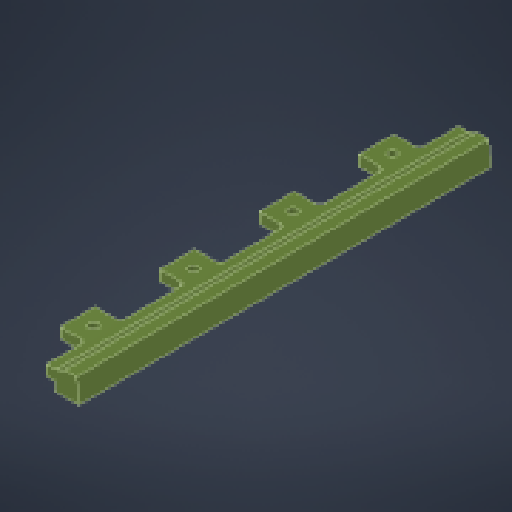
# Autodesk Inventor part: plaski_plog
Saved by Autodesk Inventor 2023 (Build 270158000, 158)
## iProperties
Created: 2024-06-19
Part Number: plaski_plog
Material: PC/ABS Plastic
Document SubType Name: Modeling
Designer: szymo
Density: 1.1 g/cm^3
Appearance: Dark Olive
Mass: 23.2841 g
Surface Area: 101.304 cm^2
Volume: 21.1673 cm^3
Author: szymo
Autodesk Inventor part; units mm, degrees
ref_plane "YZ Plane" through (0, 0, 0) normal (1, 0, 0) x (0, 1, 0)
ref_plane "XZ Plane" through (0, 0, 0) normal (0, 1, 0) x (-1, 0, 0)
sketch "Sketch1" plane through (0, 0, 0) normal (0, 0, 1) x (1, 0, 0)
  line L0 (-60.5213, -2.6863) -> (-60.5213, -7.1863) projected
  line L1 (-69.5213, -2.6863) -> (-60.5213, -2.6863) projected
  line L2 (-69.5213, -7.1863) -> (-69.5213, -2.6863) projected
  line L3 (-60.5213, -7.1863) -> (-69.5213, -7.1863) projected
  line L4 (-60.5213, -7.1863) -> (-58.5213, -7.1863) projected
  line L5 (-58.5213, -2.6863) -> (-60.5213, -2.6863) projected
  line L6 (-58.5213, -10.6863) -> (-54.5213, -10.6863) projected
  line L7 (-54.5213, -10.6863) -> (-54.5213, -7.1863) projected
  line L8 (-58.5213, -7.1863) -> (-54.5213, -7.1863) projected
  line L9 (-58.5213, -10.6863) -> (-58.5213, -7.1863) projected
  line L10 (-58.5213, -2.6863) -> (-58.5213, -7.1863) projected
  line L11 (-58.5213, -7.1863) -> (-54.5213, -7.1863) projected
  line L12 (-54.5213, -7.1863) -> (-54.5213, -10.6863) projected
  line L13 (-54.5213, -10.6863) -> (-40.5213, -10.6863) projected
  line L14 (-40.5213, -10.6863) -> (-54.5213, -1.6863) projected
  line L15 (-54.5213, -1.6863) -> (-54.5213, -2.6863) projected
  line L16 (-54.5213, -2.6863) -> (-58.5213, -2.6863) projected
  line L17 (-58.5213, -0.9637) -> (-44.5213, -0.9637)
  line L18 (-44.5213, -0.9637) -> (-44.5213, -10.9637)
  line L19 (-44.5213, -10.9637) -> (-58.5213, -10.9637)
  line L20 (-58.5213, -10.9637) -> (-58.5213, -0.9637)
  line L21 (-69.5213, -2.6863) -> (-58.5213, -2.6863)
  line L22 (-58.5213, -2.6863) -> (-58.5213, -7.1863)
  line L23 (-58.5213, -7.1863) -> (-69.5213, -7.1863)
  line L24 (-69.5213, -7.1863) -> (-69.5213, -2.6863)
  circle A0 centre (-213.5213, 2.3137) radius 25 projected
  line L25 (-213.5213, -22.6863) -> (-44.5213, -10.9637)
  line L26 (-213.5213, -22.6863) -> (-213.5213, 2.3137)
  line L27 (-44.5213, -10.9637) -> (-40.5213, -10.6863)
  line L28 (-44.5213, -10.9637) -> (-45.5667, -0.9637)
  line L29 (-58.5213, -2.6863) -> (-54.5213, -2.6863)
  line L30 (-54.5213, -2.6863) -> (-54.5213, -0.9637)
  line L31 (-54.5213, -0.9637) -> (-58.5213, -0.9637)
  line L32 (-58.5213, -0.9637) -> (-58.5213, -2.6863)
  line L33 (-54.5213, -2.6863) -> (-50.5667, -0.9637)
  line L34 (-54.5213, -10.6863) -> (-54.5213, -10.9637)
  point P0 (0, 0)
  point P1 (-53.594, -2.2824)
  point P2 (-44.5503, -10.6863)
  dimension "d0" = 14
  dimension "d1" = 10
  dimension "d3" = 88
  dimension "d15" = 5
  dimension "d16" = 23.537
  constraints: 36 end point, 6 parallel, 5 point on line, 4 perpendicular, 3 horizontal, 1 collinear, 1 vertical, 1 vertical alignment, 1 other
  measures "d0" distance of L18.end L19.end
  measures "d1" distance of L17.end L18.end
  measures "d3" angle of L25 L28
  measures "d15" distance of L33.end L28.end
  measures "d16" angle of L29 L33
extrude "Extrusion1" add sketch "Sketch1" along normal mid plane 178 contours L16 L33 L14 L28 L13 L7 L8 L10 | L33 L17 L28 L14 | L13 L28 L19 L34
sketch "Sketch2" plane through (-58.5213, -2.6863, 89) normal (0, 1, 0) x (1, 0, 0)
  circle A0 centre (-4, 67.5) radius 1.2295 projected
  circle A1 centre (-4, 153.5) radius 1.2295 projected
  circle A2 centre (-4, 110.5) radius 1.2295 projected
  circle A3 centre (-4, 24.5) radius 1.2295 projected
  line L0 (-2, 161) -> (-11, 161) projected
  line L1 (-11, 161) -> (-11, 146) projected
  line L2 (-11, 146) -> (-2, 146) projected
  arc A4 (0, 144) -> (-2, 146) centre (-2, 144) ccw projected
  line L3 (0, 144) -> (0, 120) projected
  arc A5 (-2, 118) -> (0, 120) centre (-2, 120) ccw projected
  line L4 (-2, 118) -> (-11, 118) projected
  line L5 (-11, 118) -> (-11, 103) projected
  line L6 (-11, 103) -> (-2, 103) projected
  arc A6 (0, 101) -> (-2, 103) centre (-2, 101) ccw projected
  line L7 (0, 101) -> (0, 77) projected
  arc A7 (-2, 75) -> (0, 77) centre (-2, 77) ccw projected
  line L8 (-2, 75) -> (-11, 75) projected
  line L9 (-11, 75) -> (-11, 60) projected
  line L10 (-11, 60) -> (-2, 60) projected
  arc A8 (0, 58) -> (-2, 60) centre (-2, 58) ccw projected
  line L11 (0, 58) -> (0, 34) projected
  arc A9 (-2, 32) -> (0, 34) centre (-2, 34) ccw projected
  line L12 (-2, 32) -> (-11, 32) projected
  line L13 (-11, 32) -> (-11, 17) projected
  line L14 (-11, 17) -> (-2, 17) projected
  arc A10 (0, 15) -> (-2, 17) centre (-2, 15) ccw projected
  line L15 (0, 15) -> (0, 0) projected
  line L16 (4, 0) -> (0, 0) projected
  line L17 (4, 178) -> (4, 0) projected
  line L18 (4, 178) -> (0, 178) projected
  line L19 (0, 178) -> (0, 163) projected
  arc A11 (-2, 161) -> (0, 163) centre (-2, 163) ccw projected
  line L20 (0, 178) -> (0, 0) projected
  point P0 (58.5213, 89)
  constraints: 1 other
ref_plane "Work Plane1" through (-69.5213, -7.1863, -89) normal (0, -1, 0) x (1, 0, 0)
extrude "Extrusion2" add sketch "Sketch2" against normal up to surface (4.5 mm away) contours A0 | A1 | A2 | A3 | A11 L20 A4 L2 L1 L0 | L20 A6 L6 L5 L4 A5 | L20 A8 L10 L9 L8 A7 | A10 L14 L13 L12 A9 L20
sketch "Sketch3" plane through (-69.5213, -7.1863, -57) normal (0, -1, 0) x (1, 0, 0)
  circle A0 centre (7, 78.5) radius 1.2295 projected
  circle A1 centre (7, -7.5) radius 1.2295 projected
  circle A2 centre (7, 35.5) radius 1.2295 projected
  circle A3 centre (7, 121.5) radius 1.2295 projected
  line L0 (9, -15) -> (0, -15) projected
  line L1 (0, -15) -> (0, 0) projected
  line L2 (0, 0) -> (9, 0) projected
  arc A4 (9, 0) -> (11, 2) centre (9, 2) ccw projected
  line L3 (11, 2) -> (11, 26) projected
  arc A5 (11, 26) -> (9, 28) centre (9, 26) ccw projected
  line L4 (9, 28) -> (0, 28) projected
  line L5 (0, 28) -> (0, 43) projected
  line L6 (0, 43) -> (9, 43) projected
  arc A6 (9, 43) -> (11, 45) centre (9, 45) ccw projected
  line L7 (11, 45) -> (11, 69) projected
  arc A7 (11, 69) -> (9, 71) centre (9, 69) ccw projected
  line L8 (9, 71) -> (0, 71) projected
  line L9 (0, 71) -> (0, 86) projected
  line L10 (0, 86) -> (9, 86) projected
  arc A8 (9, 86) -> (11, 88) centre (9, 88) ccw projected
  line L11 (11, 88) -> (11, 112) projected
  arc A9 (11, 112) -> (9, 114) centre (9, 112) ccw projected
  line L12 (9, 114) -> (0, 114) projected
  line L13 (0, 114) -> (0, 129) projected
  line L14 (0, 129) -> (9, 129) projected
  arc A10 (9, 129) -> (11, 131) centre (9, 131) ccw projected
  line L15 (11, 131) -> (11, 146) projected
  line L16 (15, 146) -> (11, 146) projected
  line L17 (15, -32) -> (15, 146) projected
  line L18 (15, -32) -> (11, -32) projected
  line L19 (11, -32) -> (11, -17) projected
  arc A11 (11, -17) -> (9, -15) centre (9, -17) ccw projected
  point P0 (69.5213, 57)
  constraints: 4 coincident
hole "Hole1" at (-62.5213, -7.1863, -64.5) at (-62.5213, -7.1863, -21.5) at (-62.5213, -7.1863, 21.5) at (-62.5213, -7.1863, 64.5) direction (0, 1, 0) diameter 3.9 depth 4.5 counterbore diameter 4.6 counterbore depth 0.75
body "Solid1"
